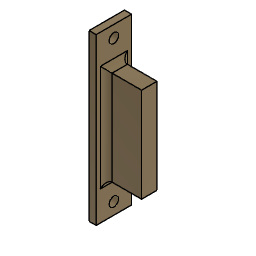
Manilla v2 (Autodesk Fusion 360 design; units mm, degrees)
Autodesk Fusion 360 part; units mm, degrees
sketch "Boceto1" plane through (0, 0, 0) normal (1, 0, 0) x (0, 1, 0)
  line L0 (7.5, 35) -> (-7.5, 35)
  line L1 (-7.5, 35) -> (-7.5, -35)
  line L2 (-7.5, -35) -> (7.5, -35)
  line L3 (7.5, -35) -> (7.5, 35)
  line L4 (7.5, 35) -> (-7.5, -35) construction
  line L5 (-7.5, 35) -> (7.5, -35) construction
  circle A0 centre (0, 30) radius 2
  circle A1 centre (0, -30) radius 2
  line L6 (0, 35) -> (0, -35) construction
  dimension "d1" = 15
  dimension "d2" = 70
  dimension "d3" = 4
  dimension "d4" = 4
  dimension "d5" = 60
  dimension "d6" = 30
  constraint horizontal L0
  constraint perpendicular L0 L1
  constraint parallel L0 L2
  constraint parallel L1 L3
  constraint coincident L4 origin
  constraint coincident L5 origin
  constraint midpoint L0 L6.start
  constraint midpoint L2 L6.end
  constraint coincident A1.centre L6
  constraint coincident A0.centre L6
  measures "d1" distance of L1.end L2.end
  measures "d2" distance of L0.end L1.end
  measures "d3" diameter of A0
  measures "d4" diameter of A1
  measures "d5" distance of A0.centre A1.centre
  measures "d6" distance of origin A1.centre
extrude "Extruir1" add sketch "Boceto1" along normal blind 3
sketch "Boceto2" plane through (3, 0, 0) normal (1, 0, 0) x (0, 1, 0)
  circle A0 centre (0, 30) radius 2
  circle A1 centre (0, -30) radius 2
  line L0 (7.5, -35) -> (7.5, 35)
  line L1 (7.5, 35) -> (-7.5, 35)
  line L2 (-7.5, 35) -> (-7.5, -35)
  line L3 (-7.5, -35) -> (7.5, -35)
  line L4 (3.25, 20) -> (-3.25, 20)
  line L5 (-3.25, 20) -> (-3.25, -20)
  line L6 (-3.25, -20) -> (3.25, -20)
  line L7 (3.25, -20) -> (3.25, 20)
  line L8 (3.25, 20) -> (-3.25, -20) construction
  line L9 (-3.25, 20) -> (3.25, -20) construction
  dimension "d9" = 6.5
  dimension "d10" = 40
  constraint horizontal L4
  constraint perpendicular L4 L5
  constraint parallel L4 L6
  constraint parallel L5 L7
  constraint coincident L8 origin
  constraint coincident L9 origin
  measures "d9" distance of L5.end L6.end
  measures "d10" distance of L4.end L5.end
extrude "Extruir2" add sketch "Boceto2" along normal blind 15 contours L4 L5 L6 L7
fillet "Empalme1" radius 2.5 4 edges at (3, 3.25, 0) (3, 0, -20) (3, -3.25, 0) (3, 0, 20)
